Autodesk Inventor part; units mm, degrees
(part 2 of 3)
sketch "Sketch58" plane through (4600, 2900, -5000) normal (1, 0, 0) x (0, 0, -1)
  line L0 (-8412.2457, 741.5985) -> (-6687.7543, 741.5985) construction
  line L1 (-6687.7543, 741.5985) -> (-6687.7543, 358.4015) construction
  line L2 (-6687.7543, 358.4015) -> (-8412.2457, 358.4015) construction
  line L3 (-8412.2457, 358.4015) -> (-8412.2457, 741.5985) construction
  line L4 (-5750, 1200) -> (-9350, 1200) projected
  line L5 (-9350, 1200) -> (-9350, -100) projected
  line L6 (-3626.6683, 741.5985) -> (-1273.3317, 741.5985) construction
  line L7 (-1273.3317, 741.5985) -> (-1273.3317, 358.4015) construction
  line L8 (-1273.3317, 358.4015) -> (-3626.6683, 358.4015) construction
  line L9 (-3626.6683, 358.4015) -> (-3626.6683, 741.5985) construction
  line L10 (-4250, 1200) -> (-650, 1200) projected
  line L11 (-4250, -100) -> (-4250, 1200) projected
  spline S0 degree 2 poles (-8269.7933, 567.8079) (-8269.7933, 547.265) (-8286.4465, 514.2018) (-8300.4254, 504.9635) knots 0 0 0 1 2 2 2
  spline S1 degree 2 poles (-8300.4254, 504.9635) (-8311.8517, 497.7917) (-8335.312, 492.9295) (-8353.5453, 492.9295) knots 0 0 0 1 2 2 2
  line L12 (-8353.5453, 492.9295) -> (-8388.0672, 492.9295)
  line L13 (-8388.0672, 492.9295) -> (-8388.0672, 642.9295)
  line L14 (-8388.0672, 642.9295) -> (-8353.91, 642.9295)
  spline S2 degree 2 poles (-8353.91, 642.9295) (-8332.7593, 642.9295) (-8308.6912, 636.6086) (-8300.1823, 631.017) knots 0 0 0 1 2 2 2
  spline S3 degree 2 poles (-8300.1823, 631.017) (-8285.7171, 621.4141) (-8269.7933, 589.688) (-8269.7933, 567.8079) knots 0 0 0 1 2 2 2
  spline S4 degree 2 poles (-8290.5794, 568.0511) (-8290.5794, 585.312) (-8302.0056, 609.7447) (-8313.3103, 616.6734) knots 0 0 0 1 2 2 2
  spline S5 degree 2 poles (-8313.3103, 616.6734) (-8321.333, 621.4141) (-8339.4449, 625.6686) (-8352.9376, 625.6686) knots 0 0 0 1 2 2 2
  line L15 (-8352.9376, 625.6686) -> (-8368.1321, 625.6686)
  line L16 (-8368.1321, 625.6686) -> (-8368.1321, 510.1904)
  line L17 (-8368.1321, 510.1904) -> (-8352.9376, 510.1904)
  spline S6 degree 2 poles (-8352.9376, 510.1904) (-8339.688, 510.1904) (-8319.6312, 514.4449) (-8311.487, 520.158) knots 0 0 0 1 2 2 2
  spline S7 degree 2 poles (-8311.487, 520.158) (-8301.0332, 527.2083) (-8290.5794, 550.547) (-8290.5794, 568.0511) knots 0 0 0 1 2 2 2
  spline S8 degree 2 poles (-8186.8922, 504.842) (-8189.2018, 503.1402) (-8196.9813, 497.0624) (-8200.628, 495.2391) knots 0 0 0 1 2 2 2
  spline S9 degree 2 poles (-8200.628, 495.2391) (-8205.6118, 492.5648) (-8214.9716, 489.769) (-8223.4805, 489.769) knots 0 0 0 1 2 2 2
  spline S10 degree 2 poles (-8223.4805, 489.769) (-8230.4092, 489.769) (-8242.9295, 494.9959) (-8247.6701, 499.7366) knots 0 0 0 1 2 2 2
  spline S11 degree 2 poles (-8247.6701, 499.7366) (-8252.1677, 504.3558) (-8257.6377, 517.97) (-8257.6377, 525.5065) knots 0 0 0 1 2 2 2
  spline S12 degree 2 poles (-8257.6377, 525.5065) (-8257.6377, 537.1759) (-8247.7917, 553.7075) (-8237.0948, 558.4481) knots 0 0 0 1 2 2 2
  spline S13 degree 2 poles (-8237.0948, 558.4481) (-8227.6134, 562.8242) (-8201.8436, 566.1062) (-8186.8922, 566.9571) knots 0 0 0 1 2 2 2
  line L18 (-8186.8922, 566.9571) -> (-8186.8922, 570.6037)
  spline S14 degree 2 poles (-8186.8922, 570.6037) (-8186.8922, 577.1677) (-8190.9035, 585.312) (-8194.5502, 587.6216) knots 0 0 0 1 2 2 2
  spline S15 degree 2 poles (-8194.5502, 587.6216) (-8198.1969, 589.9311) (-8208.6507, 591.3898) (-8214.2423, 591.3898) knots 0 0 0 1 2 2 2
  spline S16 degree 2 poles (-8214.2423, 591.3898) (-8220.8063, 591.3898) (-8238.5535, 587.5) (-8247.427, 583.7318) knots 0 0 0 1 2 2 2
  line L19 (-8247.427, 583.7318) -> (-8248.521, 583.7318)
  line L20 (-8248.521, 583.7318) -> (-8248.521, 603.0592)
  spline S17 degree 2 poles (-8248.521, 603.0592) (-8243.2941, 604.5178) (-8223.7236, 608.1645) (-8214.1207, 608.1645) knots 0 0 0 1 2 2 2
  spline S18 degree 2 poles (-8214.1207, 608.1645) (-8202.4513, 608.1645) (-8186.5275, 604.5178) (-8180.2066, 599.7771) knots 0 0 0 1 2 2 2
  spline S19 degree 2 poles (-8180.2066, 599.7771) (-8174.0073, 595.158) (-8167.9295, 580.4498) (-8167.9295, 569.8744) knots 0 0 0 1 2 2 2
  line L21 (-8167.9295, 569.8744) -> (-8167.9295, 492.9295)
  line L22 (-8167.9295, 492.9295) -> (-8186.8922, 492.9295)
  line L23 (-8186.8922, 492.9295) -> (-8186.8922, 504.842)
  line L24 (-8186.8922, 520.6442) -> (-8186.8922, 551.8841)
  spline S20 degree 2 poles (-8186.8922, 551.8841) (-8193.6993, 551.2763) (-8214.2423, 549.2099) (-8220.6847, 547.265) knots 0 0 0 1 2 2 2
  spline S21 degree 2 poles (-8220.6847, 547.265) (-8228.2212, 544.9554) (-8238.0672, 535.3525) (-8238.0672, 526.8436) knots 0 0 0 1 2 2 2
  spline S22 degree 2 poles (-8238.0672, 526.8436) (-8238.0672, 517.1191) (-8227.1272, 507.2731) (-8216.6734, 507.2731) knots 0 0 0 1 2 2 2
  spline S23 degree 2 poles (-8216.6734, 507.2731) (-8207.7998, 507.2731) (-8193.2131, 514.9311) (-8186.8922, 520.6442) knots 0 0 0 1 2 2 2
  line L25 (-8013.675, 492.9295) -> (-8013.675, 558.0835)
  spline S24 degree 2 poles (-8013.675, 558.0835) (-8013.675, 565.863) (-8014.8906, 579.1126) (-8016.8355, 582.7593) knots 0 0 0 1 2 2 2
  spline S25 degree 2 poles (-8016.8355, 582.7593) (-8018.7804, 586.7707) (-8026.1953, 590.6605) (-8032.6377, 590.6605) knots 0 0 0 1 2 2 2
  spline S26 degree 2 poles (-8032.6377, 590.6605) (-8038.4724, 590.6605) (-8051.8436, 583.4887) (-8058.8938, 576.6815) knots 0 0 0 1 2 2 2
  spline S27 degree 2 poles (-8058.8938, 576.6815) (-8058.7723, 574.9797) (-8058.5291, 570.2391) (-8058.5291, 567.0786) knots 0 0 0 1 2 2 2
  line L26 (-8058.5291, 567.0786) -> (-8058.5291, 492.9295)
  line L27 (-8058.5291, 492.9295) -> (-8077.4919, 492.9295)
  line L28 (-8077.4919, 492.9295) -> (-8077.4919, 558.0835)
  spline S28 degree 2 poles (-8077.4919, 558.0835) (-8077.4919, 565.863) (-8078.7074, 579.1126) (-8080.6523, 582.7593) knots 0 0 0 1 2 2 2
  spline S29 degree 2 poles (-8080.6523, 582.7593) (-8082.5972, 586.7707) (-8090.0121, 590.6605) (-8096.4546, 590.6605) knots 0 0 0 1 2 2 2
  spline S30 degree 2 poles (-8096.4546, 590.6605) (-8102.5324, 590.6605) (-8116.0251, 583.0024) (-8122.346, 577.0462) knots 0 0 0 1 2 2 2
  line L29 (-8122.346, 577.0462) -> (-8122.346, 492.9295)
  line L30 (-8122.346, 492.9295) -> (-8141.3087, 492.9295)
  line L31 (-8141.3087, 492.9295) -> (-8141.3087, 605.4903)
  line L32 (-8141.3087, 605.4903) -> (-8122.346, 605.4903)
  line L33 (-8122.346, 605.4903) -> (-8122.346, 593.0916)
  spline S31 degree 2 poles (-8122.346, 593.0916) (-8114.9311, 600.5065) (-8100.3444, 608.6507) (-8091.5924, 608.6507) knots 0 0 0 1 2 2 2
  spline S32 degree 2 poles (-8091.5924, 608.6507) (-8081.6248, 608.6507) (-8066.1872, 599.534) (-8062.1758, 589.2018) knots 0 0 0 1 2 2 2
  spline S33 degree 2 poles (-8062.1758, 589.2018) (-8053.5453, 598.8047) (-8037.2569, 608.6507) (-8027.7755, 608.6507) knots 0 0 0 1 2 2 2
  spline S34 degree 2 poles (-8027.7755, 608.6507) (-8020.4821, 608.6507) (-8008.5697, 604.1532) (-8004.1936, 599.0478) knots 0 0 0 1 2 2 2
  spline S35 degree 2 poles (-8004.1936, 599.0478) (-7999.6961, 593.9425) (-7994.7123, 578.6264) (-7994.7123, 567.0786) knots 0 0 0 1 2 2 2
  line L34 (-7994.7123, 567.0786) -> (-7994.7123, 492.9295)
  line L35 (-7994.7123, 492.9295) -> (-8013.675, 492.9295)
  spline S36 degree 2 poles (-7937.4594, 489.769) (-7937.4594, 470.5632) (-7958.124, 450.3849) (-7976.2358, 450.3849) knots 0 0 0 1 2 2 2
  spline S37 degree 2 poles (-7976.2358, 450.3849) (-7979.3962, 450.3849) (-7987.1758, 450.9927) (-7990.9441, 451.6005) knots 0 0 0 1 2 2 2
  line L36 (-7990.9441, 451.6005) -> (-7990.9441, 468.6183)
  line L37 (-7990.9441, 468.6183) -> (-7989.85, 468.6183)
  spline S38 degree 2 poles (-7989.85, 468.6183) (-7987.662, 468.1321) (-7982.3136, 467.1596) (-7979.8825, 467.1596) knots 0 0 0 1 2 2 2
  spline S39 degree 2 poles (-7979.8825, 467.1596) (-7972.346, 467.1596) (-7962.5, 470.9279) (-7960.1904, 474.9392) knots 0 0 0 1 2 2 2
  spline S40 degree 2 poles (-7960.1904, 474.9392) (-7957.8808, 478.5859) (-7956.4222, 489.6475) (-7956.4222, 497.5486) knots 0 0 0 1 2 2 2
  line L38 (-7956.4222, 497.5486) -> (-7956.4222, 589.8096)
  line L39 (-7956.4222, 589.8096) -> (-7976.722, 589.8096)
  line L40 (-7976.722, 589.8096) -> (-7976.722, 605.4903)
  line L41 (-7976.722, 605.4903) -> (-7937.4594, 605.4903)
  line L42 (-7937.4594, 605.4903) -> (-7937.4594, 489.769)
  line L43 (-7937.3379, 624.2099) -> (-7958.8533, 624.2099)
  line L44 (-7958.8533, 624.2099) -> (-7958.8533, 643.9019)
  line L45 (-7958.8533, 643.9019) -> (-7937.3379, 643.9019)
  line L46 (-7937.3379, 643.9019) -> (-7937.3379, 624.2099)
  spline S41 degree 2 poles (-7847.265, 504.842) (-7849.5745, 503.1402) (-7857.3541, 497.0624) (-7861.0008, 495.2391) knots 0 0 0 1 2 2 2
  spline S42 degree 2 poles (-7861.0008, 495.2391) (-7865.9846, 492.5648) (-7875.3444, 489.769) (-7883.8533, 489.769) knots 0 0 0 1 2 2 2
  spline S43 degree 2 poles (-7883.8533, 489.769) (-7890.782, 489.769) (-7903.3022, 494.9959) (-7908.0429, 499.7366) knots 0 0 0 1 2 2 2
  spline S44 degree 2 poles (-7908.0429, 499.7366) (-7912.5405, 504.3558) (-7918.0105, 517.97) (-7918.0105, 525.5065) knots 0 0 0 1 2 2 2
  spline S45 degree 2 poles (-7918.0105, 525.5065) (-7918.0105, 537.1759) (-7908.1645, 553.7075) (-7897.4676, 558.4481) knots 0 0 0 1 2 2 2
  spline S46 degree 2 poles (-7897.4676, 558.4481) (-7887.9862, 562.8242) (-7862.2163, 566.1062) (-7847.265, 566.9571) knots 0 0 0 1 2 2 2
  line L47 (-7847.265, 566.9571) -> (-7847.265, 570.6037)
  spline S47 degree 2 poles (-7847.265, 570.6037) (-7847.265, 577.1677) (-7851.2763, 585.312) (-7854.923, 587.6216) knots 0 0 0 1 2 2 2
  spline S48 degree 2 poles (-7854.923, 587.6216) (-7858.5697, 589.9311) (-7869.0235, 591.3898) (-7874.615, 591.3898) knots 0 0 0 1 2 2 2
  spline S49 degree 2 poles (-7874.615, 591.3898) (-7881.1791, 591.3898) (-7898.9262, 587.5) (-7907.7998, 583.7318) knots 0 0 0 1 2 2 2
  line L48 (-7907.7998, 583.7318) -> (-7908.8938, 583.7318)
  line L49 (-7908.8938, 583.7318) -> (-7908.8938, 603.0592)
  spline S50 degree 2 poles (-7908.8938, 603.0592) (-7903.6669, 604.5178) (-7884.0964, 608.1645) (-7874.4935, 608.1645) knots 0 0 0 1 2 2 2
  spline S51 degree 2 poles (-7874.4935, 608.1645) (-7862.8241, 608.1645) (-7846.9003, 604.5178) (-7840.5794, 599.7771) knots 0 0 0 1 2 2 2
  spline S52 degree 2 poles (-7840.5794, 599.7771) (-7834.38, 595.158) (-7828.3022, 580.4498) (-7828.3022, 569.8744) knots 0 0 0 1 2 2 2
  line L50 (-7828.3022, 569.8744) -> (-7828.3022, 492.9295)
  line L51 (-7828.3022, 492.9295) -> (-7847.265, 492.9295)
  line L52 (-7847.265, 492.9295) -> (-7847.265, 504.842)
  line L53 (-7847.265, 520.6442) -> (-7847.265, 551.8841)
  spline S53 degree 2 poles (-7847.265, 551.8841) (-7854.0721, 551.2763) (-7874.615, 549.2099) (-7881.0575, 547.265) knots 0 0 0 1 2 2 2
  spline S54 degree 2 poles (-7881.0575, 547.265) (-7888.594, 544.9554) (-7898.44, 535.3525) (-7898.44, 526.8436) knots 0 0 0 1 2 2 2
  spline S55 degree 2 poles (-7898.44, 526.8436) (-7898.44, 517.1191) (-7887.5, 507.2731) (-7877.0462, 507.2731) knots 0 0 0 1 2 2 2
  spline S56 degree 2 poles (-7877.0462, 507.2731) (-7868.1726, 507.2731) (-7853.5859, 514.9311) (-7847.265, 520.6442) knots 0 0 0 1 2 2 2
  line L54 (-7713.3103, 492.9295) -> (-7732.2731, 492.9295)
  line L55 (-7732.2731, 492.9295) -> (-7732.2731, 557.111)
  spline S57 degree 2 poles (-7732.2731, 557.111) (-7732.2731, 564.8906) (-7733.7317, 578.2618) (-7735.9197, 582.2731) knots 0 0 0 1 2 2 2
  spline S58 degree 2 poles (-7735.9197, 582.2731) (-7738.2293, 586.5276) (-7746.4951, 590.6605) (-7753.5453, 590.6605) knots 0 0 0 1 2 2 2
  spline S59 degree 2 poles (-7753.5453, 590.6605) (-7760.5956, 590.6605) (-7775.547, 583.124) (-7782.7188, 577.0462) knots 0 0 0 1 2 2 2
  line L56 (-7782.7188, 577.0462) -> (-7782.7188, 492.9295)
  line L57 (-7782.7188, 492.9295) -> (-7801.6815, 492.9295)
  line L58 (-7801.6815, 492.9295) -> (-7801.6815, 605.4903)
  line L59 (-7801.6815, 605.4903) -> (-7782.7188, 605.4903)
  line L60 (-7782.7188, 605.4903) -> (-7782.7188, 592.97)
  spline S60 degree 2 poles (-7782.7188, 592.97) (-7774.2099, 600.628) (-7757.7998, 608.6507) (-7748.5616, 608.6507) knots 0 0 0 1 2 2 2
  spline S61 degree 2 poles (-7748.5616, 608.6507) (-7732.03, 608.6507) (-7713.3103, 586.7707) (-7713.3103, 565.9846) knots 0 0 0 1 2 2 2
  line L61 (-7713.3103, 565.9846) -> (-7713.3103, 492.9295)
  line L62 (-7525.1418, 492.9295) -> (-7629.923, 492.9295)
  line L63 (-7629.923, 492.9295) -> (-7629.923, 511.5276)
  line L64 (-7629.923, 511.5276) -> (-7549.6961, 625.1823)
  line L65 (-7549.6961, 625.1823) -> (-7626.2763, 625.1823)
  line L66 (-7626.2763, 625.1823) -> (-7626.2763, 642.9295)
  line L67 (-7626.2763, 642.9295) -> (-7527.2082, 642.9295)
  line L68 (-7527.2082, 642.9295) -> (-7527.2082, 624.9392)
  line L69 (-7527.2082, 624.9392) -> (-7608.286, 510.6767)
  line L70 (-7608.286, 510.6767) -> (-7525.1418, 510.6767)
  line L71 (-7525.1418, 510.6767) -> (-7525.1418, 492.9295)
  spline S62 degree 2 poles (-7458.0429, 490.3768) (-7485.0283, 490.3768) (-7514.688, 520.6442) (-7514.688, 548.6021) knots 0 0 0 1 2 2 2
  spline S63 degree 2 poles (-7514.688, 548.6021) (-7514.688, 576.0737) (-7485.8792, 608.6507) (-7462.662, 608.6507) knots 0 0 0 1 2 2 2
  spline S64 degree 2 poles (-7462.662, 608.6507) (-7452.2082, 608.6507) (-7436.0413, 602.5729) (-7430.0851, 596.1305) knots 0 0 0 1 2 2 2
  spline S65 degree 2 poles (-7430.0851, 596.1305) (-7424.0073, 589.688) (-7417.5648, 571.09) (-7417.5648, 557.5972) knots 0 0 0 1 2 2 2
  line L72 (-7417.5648, 557.5972) -> (-7417.5648, 547.265)
  line L73 (-7417.5648, 547.265) -> (-7495.4821, 547.265)
  spline S66 degree 2 poles (-7495.4821, 547.265) (-7495.4821, 527.6945) (-7475.7901, 506.9084) (-7458.286, 506.9084) knots 0 0 0 1 2 2 2
  spline S67 degree 2 poles (-7458.286, 506.9084) (-7452.0867, 506.9084) (-7440.0526, 509.7042) (-7435.1904, 511.8922) knots 0 0 0 1 2 2 2
  spline S68 degree 2 poles (-7435.1904, 511.8922) (-7430.0851, 514.3233) (-7423.0348, 518.5778) (-7420.7253, 520.5227) knots 0 0 0 1 2 2 2
  line L74 (-7420.7253, 520.5227) -> (-7419.6312, 520.5227)
  line L75 (-7419.6312, 520.5227) -> (-7419.6312, 499.8582)
  spline S69 degree 2 poles (-7419.6312, 499.8582) (-7422.9133, 498.5211) (-7432.8808, 494.6313) (-7436.7706, 493.5373) knots 0 0 0 1 2 2 2
  spline S70 degree 2 poles (-7436.7706, 493.5373) (-7442.2406, 491.9571) (-7451.2358, 490.3768) (-7458.0429, 490.3768) knots 0 0 0 1 2 2 2
  spline S71 degree 2 poles (-7436.0413, 561.7301) (-7436.2844, 569.3882) (-7439.4449, 580.5713) (-7442.4838, 584.3395) knots 0 0 0 1 2 2 2
  spline S72 degree 2 poles (-7442.4838, 584.3395) (-7445.7658, 588.594) (-7456.098, 593.0916) (-7463.756, 593.0916) knots 0 0 0 1 2 2 2
  spline S73 degree 2 poles (-7463.756, 593.0916) (-7471.2925, 593.0916) (-7481.8679, 588.594) (-7486.2439, 584.218) knots 0 0 0 1 2 2 2
  spline S74 degree 2 poles (-7486.2439, 584.218) (-7490.4983, 579.7204) (-7494.8744, 568.9019) (-7495.4821, 561.7301) knots 0 0 0 1 2 2 2
  line L76 (-7495.4821, 561.7301) -> (-7436.0413, 561.7301)
  line L77 (-7379.0316, 492.9295) -> (-7397.9943, 492.9295)
  line L78 (-7397.9943, 492.9295) -> (-7397.9943, 649.6151)
  line L79 (-7397.9943, 649.6151) -> (-7379.0316, 649.6151)
  line L80 (-7379.0316, 649.6151) -> (-7379.0316, 492.9295)
  spline S75 degree 2 poles (-7302.3298, 490.3768) (-7329.3152, 490.3768) (-7358.9748, 520.6442) (-7358.9748, 548.6021) knots 0 0 0 1 2 2 2
  spline S76 degree 2 poles (-7358.9748, 548.6021) (-7358.9748, 576.0737) (-7330.1661, 608.6507) (-7306.9489, 608.6507) knots 0 0 0 1 2 2 2
  spline S77 degree 2 poles (-7306.9489, 608.6507) (-7296.4951, 608.6507) (-7280.3282, 602.5729) (-7274.3719, 596.1305) knots 0 0 0 1 2 2 2
  spline S78 degree 2 poles (-7274.3719, 596.1305) (-7268.2941, 589.688) (-7261.8517, 571.09) (-7261.8517, 557.5972) knots 0 0 0 1 2 2 2
  line L81 (-7261.8517, 557.5972) -> (-7261.8517, 547.265)
  line L82 (-7261.8517, 547.265) -> (-7339.769, 547.265)
  spline S79 degree 2 poles (-7339.769, 547.265) (-7339.769, 527.6945) (-7320.077, 506.9084) (-7302.5729, 506.9084) knots 0 0 0 1 2 2 2
  spline S80 degree 2 poles (-7302.5729, 506.9084) (-7296.3736, 506.9084) (-7284.3395, 509.7042) (-7279.4773, 511.8922) knots 0 0 0 1 2 2 2
  spline S81 degree 2 poles (-7279.4773, 511.8922) (-7274.3719, 514.3233) (-7267.3217, 518.5778) (-7265.0121, 520.5227) knots 0 0 0 1 2 2 2
  line L83 (-7265.0121, 520.5227) -> (-7263.9181, 520.5227)
  line L84 (-7263.9181, 520.5227) -> (-7263.9181, 499.8582)
  spline S82 degree 2 poles (-7263.9181, 499.8582) (-7267.2001, 498.5211) (-7277.1677, 494.6313) (-7281.0575, 493.5373) knots 0 0 0 1 2 2 2
  spline S83 degree 2 poles (-7281.0575, 493.5373) (-7286.5275, 491.9571) (-7295.5227, 490.3768) (-7302.3298, 490.3768) knots 0 0 0 1 2 2 2
  spline S84 degree 2 poles (-7280.3282, 561.7301) (-7280.5713, 569.3882) (-7283.7317, 580.5713) (-7286.7706, 584.3395) knots 0 0 0 1 2 2 2
  spline S85 degree 2 poles (-7286.7706, 584.3395) (-7290.0526, 588.594) (-7300.3849, 593.0916) (-7308.0429, 593.0916) knots 0 0 0 1 2 2 2
  spline S86 degree 2 poles (-7308.0429, 593.0916) (-7315.5794, 593.0916) (-7326.1547, 588.594) (-7330.5308, 584.218) knots 0 0 0 1 2 2 2
  spline S87 degree 2 poles (-7330.5308, 584.218) (-7334.7852, 579.7204) (-7339.1612, 568.9019) (-7339.769, 561.7301) knots 0 0 0 1 2 2 2
  line L85 (-7339.769, 561.7301) -> (-7280.3282, 561.7301)
  line L86 (-7154.2747, 492.9295) -> (-7173.2374, 492.9295)
  line L87 (-7173.2374, 492.9295) -> (-7173.2374, 557.111)
  spline S88 degree 2 poles (-7173.2374, 557.111) (-7173.2374, 564.8906) (-7174.6961, 578.2618) (-7176.8841, 582.2731) knots 0 0 0 1 2 2 2
  spline S89 degree 2 poles (-7176.8841, 582.2731) (-7179.1936, 586.5276) (-7187.4594, 590.6605) (-7194.5097, 590.6605) knots 0 0 0 1 2 2 2
  spline S90 degree 2 poles (-7194.5097, 590.6605) (-7201.5599, 590.6605) (-7216.5113, 583.124) (-7223.6831, 577.0462) knots 0 0 0 1 2 2 2
  line L88 (-7223.6831, 577.0462) -> (-7223.6831, 492.9295)
  line L89 (-7223.6831, 492.9295) -> (-7242.6458, 492.9295)
  line L90 (-7242.6458, 492.9295) -> (-7242.6458, 605.4903)
  line L91 (-7242.6458, 605.4903) -> (-7223.6831, 605.4903)
  line L92 (-7223.6831, 605.4903) -> (-7223.6831, 592.97)
  spline S91 degree 2 poles (-7223.6831, 592.97) (-7215.1742, 600.628) (-7198.7641, 608.6507) (-7189.5259, 608.6507) knots 0 0 0 1 2 2 2
  spline S92 degree 2 poles (-7189.5259, 608.6507) (-7172.9943, 608.6507) (-7154.2747, 586.7707) (-7154.2747, 565.9846) knots 0 0 0 1 2 2 2
  line L93 (-7154.2747, 565.9846) -> (-7154.2747, 492.9295)
  spline S93 degree 2 poles (-7033.3265, 551.0332) (-7033.3265, 523.44) (-7060.0689, 489.769) (-7080.2471, 489.769) knots 0 0 0 1 2 2 2
  spline S94 degree 2 poles (-7080.2471, 489.769) (-7089.3638, 489.769) (-7102.3703, 494.2666) (-7108.6912, 498.1564) knots 0 0 0 1 2 2 2
  line L94 (-7108.6912, 498.1564) -> (-7109.9068, 492.9295)
  line L95 (-7109.9068, 492.9295) -> (-7127.6539, 492.9295)
  line L96 (-7127.6539, 492.9295) -> (-7127.6539, 649.6151)
  line L97 (-7127.6539, 649.6151) -> (-7108.6912, 649.6151)
  line L98 (-7108.6912, 649.6151) -> (-7108.6912, 593.6994)
  spline S95 degree 2 poles (-7108.6912, 593.6994) (-7101.5194, 600.1418) (-7084.8663, 608.6507) (-7074.2909, 608.6507) knots 0 0 0 1 2 2 2
  spline S96 degree 2 poles (-7074.2909, 608.6507) (-7055.2066, 608.6507) (-7033.3265, 578.1402) (-7033.3265, 551.0332) knots 0 0 0 1 2 2 2
  spline S97 degree 2 poles (-7052.8971, 549.5746) (-7052.8971, 569.7528) (-7065.1742, 590.6605) (-7078.7885, 590.6605) knots 0 0 0 1 2 2 2
  spline S98 degree 2 poles (-7078.7885, 590.6605) (-7086.4465, 590.6605) (-7102.2488, 583.3671) (-7108.6912, 577.7755) knots 0 0 0 1 2 2 2
  line L99 (-7108.6912, 577.7755) -> (-7108.6912, 513.2293)
  spline S99 degree 2 poles (-7108.6912, 513.2293) (-7101.5194, 509.7042) (-7090.4578, 506.7869) (-7083.8938, 506.7869) knots 0 0 0 1 2 2 2
  spline S100 degree 2 poles (-7083.8938, 506.7869) (-7069.4287, 506.7869) (-7052.8971, 527.3298) (-7052.8971, 549.5746) knots 0 0 0 1 2 2 2
  spline S101 degree 2 poles (-6950.9116, 504.842) (-6953.2212, 503.1402) (-6961.0008, 497.0624) (-6964.6475, 495.2391) knots 0 0 0 1 2 2 2
  spline S102 degree 2 poles (-6964.6475, 495.2391) (-6969.6312, 492.5648) (-6978.9911, 489.769) (-6987.5, 489.769) knots 0 0 0 1 2 2 2
  spline S103 degree 2 poles (-6987.5, 489.769) (-6994.4287, 489.769) (-7006.9489, 494.9959) (-7011.6896, 499.7366) knots 0 0 0 1 2 2 2
  spline S104 degree 2 poles (-7011.6896, 499.7366) (-7016.1872, 504.3558) (-7021.6572, 517.97) (-7021.6572, 525.5065) knots 0 0 0 1 2 2 2
  spline S105 degree 2 poles (-7021.6572, 525.5065) (-7021.6572, 537.1759) (-7011.8112, 553.7075) (-7001.1142, 558.4481) knots 0 0 0 1 2 2 2
  spline S106 degree 2 poles (-7001.1142, 558.4481) (-6991.6329, 562.8242) (-6965.863, 566.1062) (-6950.9116, 566.9571) knots 0 0 0 1 2 2 2
  line L100 (-6950.9116, 566.9571) -> (-6950.9116, 570.6037)
  spline S107 degree 2 poles (-6950.9116, 570.6037) (-6950.9116, 577.1677) (-6954.923, 585.312) (-6958.5697, 587.6216) knots 0 0 0 1 2 2 2
  spline S108 degree 2 poles (-6958.5697, 587.6216) (-6962.2163, 589.9311) (-6972.6701, 591.3898) (-6978.2617, 591.3898) knots 0 0 0 1 2 2 2
  spline S109 degree 2 poles (-6978.2617, 591.3898) (-6984.8257, 591.3898) (-7002.5729, 587.5) (-7011.4465, 583.7318) knots 0 0 0 1 2 2 2
  line L101 (-7011.4465, 583.7318) -> (-7012.5405, 583.7318)
  line L102 (-7012.5405, 583.7318) -> (-7012.5405, 603.0592)
  spline S110 degree 2 poles (-7012.5405, 603.0592) (-7007.3136, 604.5178) (-6987.7431, 608.1645) (-6978.1402, 608.1645) knots 0 0 0 1 2 2 2
  spline S111 degree 2 poles (-6978.1402, 608.1645) (-6966.4708, 608.1645) (-6950.547, 604.5178) (-6944.2261, 599.7771) knots 0 0 0 1 2 2 2
  spline S112 degree 2 poles (-6944.2261, 599.7771) (-6938.0267, 595.158) (-6931.9489, 580.4498) (-6931.9489, 569.8744) knots 0 0 0 1 2 2 2
  line L103 (-6931.9489, 569.8744) -> (-6931.9489, 492.9295)
  line L104 (-6931.9489, 492.9295) -> (-6950.9116, 492.9295)
  line L105 (-6950.9116, 492.9295) -> (-6950.9116, 504.842)
  line L106 (-6950.9116, 520.6442) -> (-6950.9116, 551.8841)
  spline S113 degree 2 poles (-6950.9116, 551.8841) (-6957.7188, 551.2763) (-6978.2617, 549.2099) (-6984.7042, 547.265) knots 0 0 0 1 2 2 2
  spline S114 degree 2 poles (-6984.7042, 547.265) (-6992.2406, 544.9554) (-7002.0867, 535.3525) (-7002.0867, 526.8436) knots 0 0 0 1 2 2 2
  spline S115 degree 2 poles (-7002.0867, 526.8436) (-7002.0867, 517.1191) (-6991.1466, 507.2731) (-6980.6928, 507.2731) knots 0 0 0 1 2 2 2
  spline S116 degree 2 poles (-6980.6928, 507.2731) (-6971.8193, 507.2731) (-6957.2325, 514.9311) (-6950.9116, 520.6442) knots 0 0 0 1 2 2 2
  spline S117 degree 2 poles (-6811.0008, 551.0332) (-6811.0008, 523.44) (-6837.7431, 489.769) (-6857.9214, 489.769) knots 0 0 0 1 2 2 2
  spline S118 degree 2 poles (-6857.9214, 489.769) (-6867.0381, 489.769) (-6880.0445, 494.2666) (-6886.3654, 498.1564) knots 0 0 0 1 2 2 2
  line L107 (-6886.3654, 498.1564) -> (-6887.581, 492.9295)
  line L108 (-6887.581, 492.9295) -> (-6905.3282, 492.9295)
  line L109 (-6905.3282, 492.9295) -> (-6905.3282, 649.6151)
  line L110 (-6905.3282, 649.6151) -> (-6886.3654, 649.6151)
  line L111 (-6886.3654, 649.6151) -> (-6886.3654, 593.6994)
  spline S119 degree 2 poles (-6886.3654, 593.6994) (-6879.1936, 600.1418) (-6862.5405, 608.6507) (-6851.9651, 608.6507) knots 0 0 0 1 2 2 2
  spline S120 degree 2 poles (-6851.9651, 608.6507) (-6832.8808, 608.6507) (-6811.0008, 578.1402) (-6811.0008, 551.0332) knots 0 0 0 1 2 2 2
  spline S121 degree 2 poles (-6830.5713, 549.5746) (-6830.5713, 569.7528) (-6842.8484, 590.6605) (-6856.4627, 590.6605) knots 0 0 0 1 2 2 2
  spline S122 degree 2 poles (-6856.4627, 590.6605) (-6864.1207, 590.6605) (-6879.923, 583.3671) (-6886.3654, 577.7755) knots 0 0 0 1 2 2 2
  line L112 (-6886.3654, 577.7755) -> (-6886.3654, 513.2293)
  spline S123 degree 2 poles (-6886.3654, 513.2293) (-6879.1936, 509.7042) (-6868.1321, 506.7869) (-6861.568, 506.7869) knots 0 0 0 1 2 2 2
  spline S124 degree 2 poles (-6861.568, 506.7869) (-6847.1029, 506.7869) (-6830.5713, 527.3298) (-6830.5713, 549.5746) knots 0 0 0 1 2 2 2
  spline S125 degree 2 poles (-6728.5859, 504.842) (-6730.8954, 503.1402) (-6738.675, 497.0624) (-6742.3217, 495.2391) knots 0 0 0 1 2 2 2
  spline S126 degree 2 poles (-6742.3217, 495.2391) (-6747.3055, 492.5648) (-6756.6653, 489.769) (-6765.1742, 489.769) knots 0 0 0 1 2 2 2
  spline S127 degree 2 poles (-6765.1742, 489.769) (-6772.1029, 489.769) (-6784.6231, 494.9959) (-6789.3638, 499.7366) knots 0 0 0 1 2 2 2
  spline S128 degree 2 poles (-6789.3638, 499.7366) (-6793.8614, 504.3558) (-6799.3314, 517.97) (-6799.3314, 525.5065) knots 0 0 0 1 2 2 2
  spline S129 degree 2 poles (-6799.3314, 525.5065) (-6799.3314, 537.1759) (-6789.4854, 553.7075) (-6778.7885, 558.4481) knots 0 0 0 1 2 2 2
  spline S130 degree 2 poles (-6778.7885, 558.4481) (-6769.3071, 562.8242) (-6743.5372, 566.1062) (-6728.5859, 566.9571) knots 0 0 0 1 2 2 2
  line L113 (-6728.5859, 566.9571) -> (-6728.5859, 570.6037)
  spline S131 degree 2 poles (-6728.5859, 570.6037) (-6728.5859, 577.1677) (-6732.5972, 585.312) (-6736.2439, 587.6216) knots 0 0 0 1 2 2 2
  spline S132 degree 2 poles (-6736.2439, 587.6216) (-6739.8906, 589.9311) (-6750.3444, 591.3898) (-6755.9359, 591.3898) knots 0 0 0 1 2 2 2
  spline S133 degree 2 poles (-6755.9359, 591.3898) (-6762.5, 591.3898) (-6780.2471, 587.5) (-6789.1207, 583.7318) knots 0 0 0 1 2 2 2
  line L114 (-6789.1207, 583.7318) -> (-6790.2147, 583.7318)
  line L115 (-6790.2147, 583.7318) -> (-6790.2147, 603.0592)
  spline S134 degree 2 poles (-6790.2147, 603.0592) (-6784.9878, 604.5178) (-6765.4173, 608.1645) (-6755.8144, 608.1645) knots 0 0 0 1 2 2 2
  spline S135 degree 2 poles (-6755.8144, 608.1645) (-6744.145, 608.1645) (-6728.2212, 604.5178) (-6721.9003, 599.7771) knots 0 0 0 1 2 2 2
  spline S136 degree 2 poles (-6721.9003, 599.7771) (-6715.7009, 595.158) (-6709.6231, 580.4498) (-6709.6231, 569.8744) knots 0 0 0 1 2 2 2
  line L116 (-6709.6231, 569.8744) -> (-6709.6231, 492.9295)
  line L117 (-6709.6231, 492.9295) -> (-6728.5859, 492.9295)
  line L118 (-6728.5859, 492.9295) -> (-6728.5859, 504.842)
  line L119 (-6728.5859, 520.6442) -> (-6728.5859, 551.8841)
  spline S137 degree 2 poles (-6728.5859, 551.8841) (-6735.393, 551.2763) (-6755.9359, 549.2099) (-6762.3784, 547.265) knots 0 0 0 1 2 2 2
  spline S138 degree 2 poles (-6762.3784, 547.265) (-6769.9149, 544.9554) (-6779.7609, 535.3525) (-6779.7609, 526.8436) knots 0 0 0 1 2 2 2
  spline S139 degree 2 poles (-6779.7609, 526.8436) (-6779.7609, 517.1191) (-6768.8209, 507.2731) (-6758.3671, 507.2731) knots 0 0 0 1 2 2 2
  spline S140 degree 2 poles (-6758.3671, 507.2731) (-6749.4935, 507.2731) (-6734.9068, 514.9311) (-6728.5859, 520.6442) knots 0 0 0 1 2 2 2
  spline S141 degree 2 poles (-3169.7933, 567.8079) (-3169.7933, 547.265) (-3186.4465, 514.2018) (-3200.4254, 504.9635) knots 0 0 0 1 2 2 2
  spline S142 degree 2 poles (-3200.4254, 504.9635) (-3211.8517, 497.7917) (-3235.312, 492.9295) (-3253.5453, 492.9295) knots 0 0 0 1 2 2 2
  line L120 (-3253.5453, 492.9295) -> (-3288.0672, 492.9295)
  line L121 (-3288.0672, 492.9295) -> (-3288.0672, 642.9295)
  line L122 (-3288.0672, 642.9295) -> (-3253.91, 642.9295)
  spline S143 degree 2 poles (-3253.91, 642.9295) (-3232.7593, 642.9295) (-3208.6912, 636.6086) (-3200.1823, 631.017) knots 0 0 0 1 2 2 2
  spline S144 degree 2 poles (-3200.1823, 631.017) (-3185.7171, 621.4141) (-3169.7933, 589.688) (-3169.7933, 567.8079) knots 0 0 0 1 2 2 2
  spline S145 degree 2 poles (-3190.5794, 568.0511) (-3190.5794, 585.312) (-3202.0056, 609.7447) (-3213.3103, 616.6734) knots 0 0 0 1 2 2 2
  spline S146 degree 2 poles (-3213.3103, 616.6734) (-3221.333, 621.4141) (-3239.4449, 625.6686) (-3252.9376, 625.6686) knots 0 0 0 1 2 2 2
  line L123 (-3252.9376, 625.6686) -> (-3268.1321, 625.6686)
  line L124 (-3268.1321, 625.6686) -> (-3268.1321, 510.1904)
  line L125 (-3268.1321, 510.1904) -> (-3252.9376, 510.1904)
  spline S147 degree 2 poles (-3252.9376, 510.1904) (-3239.688, 510.1904) (-3219.6312, 514.4449) (-3211.487, 520.158) knots 0 0 0 1 2 2 2
  spline S148 degree 2 poles (-3211.487, 520.158) (-3201.0332, 527.2083) (-3190.5794, 550.547) (-3190.5794, 568.0511) knots 0 0 0 1 2 2 2
  spline S149 degree 2 poles (-3086.8922, 504.842) (-3089.2018, 503.1402) (-3096.9813, 497.0624) (-3100.628, 495.2391) knots 0 0 0 1 2 2 2
  spline S150 degree 2 poles (-3100.628, 495.2391) (-3105.6118, 492.5648) (-3114.9716, 489.769) (-3123.4805, 489.769) knots 0 0 0 1 2 2 2
  spline S151 degree 2 poles (-3123.4805, 489.769) (-3130.4092, 489.769) (-3142.9295, 494.9959) (-3147.6701, 499.7366) knots 0 0 0 1 2 2 2
  spline S152 degree 2 poles (-3147.6701, 499.7366) (-3152.1677, 504.3558) (-3157.6377, 517.97) (-3157.6377, 525.5065) knots 0 0 0 1 2 2 2
  spline S153 degree 2 poles (-3157.6377, 525.5065) (-3157.6377, 537.1759) (-3147.7917, 553.7075) (-3137.0948, 558.4481) knots 0 0 0 1 2 2 2
  spline S154 degree 2 poles (-3137.0948, 558.4481) (-3127.6134, 562.8242) (-3101.8436, 566.1062) (-3086.8922, 566.9571) knots 0 0 0 1 2 2 2
  line L126 (-3086.8922, 566.9571) -> (-3086.8922, 570.6037)
  spline S155 degree 2 poles (-3086.8922, 570.6037) (-3086.8922, 577.1677) (-3090.9035, 585.312) (-3094.5502, 587.6216) knots 0 0 0 1 2 2 2
  spline S156 degree 2 poles (-3094.5502, 587.6216) (-3098.1969, 589.9311) (-3108.6507, 591.3898) (-3114.2423, 591.3898) knots 0 0 0 1 2 2 2
  spline S157 degree 2 poles (-3114.2423, 591.3898) (-3120.8063, 591.3898) (-3138.5535, 587.5) (-3147.427, 583.7318) knots 0 0 0 1 2 2 2
  line L127 (-3147.427, 583.7318) -> (-3148.521, 583.7318)
  line L128 (-3148.521, 583.7318) -> (-3148.521, 603.0592)
  spline S158 degree 2 poles (-3148.521, 603.0592) (-3143.2941, 604.5178) (-3123.7236, 608.1645) (-3114.1207, 608.1645) knots 0 0 0 1 2 2 2
  spline S159 degree 2 poles (-3114.1207, 608.1645) (-3102.4513, 608.1645) (-3086.5275, 604.5178) (-3080.2066, 599.7771) knots 0 0 0 1 2 2 2
  spline S160 degree 2 poles (-3080.2066, 599.7771) (-3074.0073, 595.158) (-3067.9295, 580.4498) (-3067.9295, 569.8744) knots 0 0 0 1 2 2 2
  line L129 (-3067.9295, 569.8744) -> (-3067.9295, 492.9295)
  line L130 (-3067.9295, 492.9295) -> (-3086.8922, 492.9295)
  line L131 (-3086.8922, 492.9295) -> (-3086.8922, 504.842)
  line L132 (-3086.8922, 520.6442) -> (-3086.8922, 551.8841)
  spline S161 degree 2 poles (-3086.8922, 551.8841) (-3093.6993, 551.2763) (-3114.2423, 549.2099) (-3120.6847, 547.265) knots 0 0 0 1 2 2 2
  spline S162 degree 2 poles (-3120.6847, 547.265) (-3128.2212, 544.9554) (-3138.0672, 535.3525) (-3138.0672, 526.8436) knots 0 0 0 1 2 2 2
  spline S163 degree 2 poles (-3138.0672, 526.8436) (-3138.0672, 517.1191) (-3127.1272, 507.2731) (-3116.6734, 507.2731) knots 0 0 0 1 2 2 2
  spline S164 degree 2 poles (-3116.6734, 507.2731) (-3107.7998, 507.2731) (-3093.2131, 514.9311) (-3086.8922, 520.6442) knots 0 0 0 1 2 2 2
  line L133 (-2913.675, 492.9295) -> (-2913.675, 558.0835)
  spline S165 degree 2 poles (-2913.675, 558.0835) (-2913.675, 565.863) (-2914.8906, 579.1126) (-2916.8355, 582.7593) knots 0 0 0 1 2 2 2
  spline S166 degree 2 poles (-2916.8355, 582.7593) (-2918.7804, 586.7707) (-2926.1953, 590.6605) (-2932.6377, 590.6605) knots 0 0 0 1 2 2 2
  spline S167 degree 2 poles (-2932.6377, 590.6605) (-2938.4724, 590.6605) (-2951.8436, 583.4887) (-2958.8938, 576.6815) knots 0 0 0 1 2 2 2
  spline S168 degree 2 poles (-2958.8938, 576.6815) (-2958.7723, 574.9797) (-2958.5291, 570.2391) (-2958.5291, 567.0786) knots 0 0 0 1 2 2 2
  line L134 (-2958.5291, 567.0786) -> (-2958.5291, 492.9295)
  line L135 (-2958.5291, 492.9295) -> (-2977.4919, 492.9295)
  line L136 (-2977.4919, 492.9295) -> (-2977.4919, 558.0835)
  spline S169 degree 2 poles (-2977.4919, 558.0835) (-2977.4919, 565.863) (-2978.7074, 579.1126) (-2980.6523, 582.7593) knots 0 0 0 1 2 2 2
  spline S170 degree 2 poles (-2980.6523, 582.7593) (-2982.5972, 586.7707) (-2990.0121, 590.6605) (-2996.4546, 590.6605) knots 0 0 0 1 2 2 2
  spline S171 degree 2 poles (-2996.4546, 590.6605) (-3002.5324, 590.6605) (-3016.0251, 583.0024) (-3022.346, 577.0462) knots 0 0 0 1 2 2 2
  line L137 (-3022.346, 577.0462) -> (-3022.346, 492.9295)
  line L138 (-3022.346, 492.9295) -> (-3041.3087, 492.9295)
  line L139 (-3041.3087, 492.9295) -> (-3041.3087, 605.4903)
  line L140 (-3041.3087, 605.4903) -> (-3022.346, 605.4903)
  line L141 (-3022.346, 605.4903) -> (-3022.346, 593.0916)
  spline S172 degree 2 poles (-3022.346, 593.0916) (-3014.9311, 600.5065) (-3000.3444, 608.6507) (-2991.5924, 608.6507) knots 0 0 0 1 2 2 2
  spline S173 degree 2 poles (-2991.5924, 608.6507) (-2981.6248, 608.6507) (-2966.1872, 599.534) (-2962.1758, 589.2018) knots 0 0 0 1 2 2 2
  spline S174 degree 2 poles (-2962.1758, 589.2018) (-2953.5453, 598.8047) (-2937.2569, 608.6507) (-2927.7755, 608.6507) knots 0 0 0 1 2 2 2
  spline S175 degree 2 poles (-2927.7755, 608.6507) (-2920.4821, 608.6507) (-2908.5697, 604.1532) (-2904.1936, 599.0478) knots 0 0 0 1 2 2 2
  spline S176 degree 2 poles (-2904.1936, 599.0478) (-2899.6961, 593.9425) (-2894.7123, 578.6264) (-2894.7123, 567.0786) knots 0 0 0 1 2 2 2
  line L142 (-2894.7123, 567.0786) -> (-2894.7123, 492.9295)
  line L143 (-2894.7123, 492.9295) -> (-2913.675, 492.9295)
  spline S177 degree 2 poles (-2837.4594, 489.769) (-2837.4594, 470.5632) (-2858.124, 450.3849) (-2876.2358, 450.3849) knots 0 0 0 1 2 2 2
  spline S178 degree 2 poles (-2876.2358, 450.3849) (-2879.3962, 450.3849) (-2887.1758, 450.9927) (-2890.9441, 451.6005) knots 0 0 0 1 2 2 2
  line L144 (-2890.9441, 451.6005) -> (-2890.9441, 468.6183)
  line L145 (-2890.9441, 468.6183) -> (-2889.85, 468.6183)
  spline S179 degree 2 poles (-2889.85, 468.6183) (-2887.662, 468.1321) (-2882.3136, 467.1596) (-2879.8825, 467.1596) knots 0 0 0 1 2 2 2
  spline S180 degree 2 poles (-2879.8825, 467.1596) (-2872.346, 467.1596) (-2862.5, 470.9279) (-2860.1904, 474.9392) knots 0 0 0 1 2 2 2
  spline S181 degree 2 poles (-2860.1904, 474.9392) (-2857.8808, 478.5859) (-2856.4222, 489.6475) (-2856.4222, 497.5486) knots 0 0 0 1 2 2 2
  line L146 (-2856.4222, 497.5486) -> (-2856.4222, 589.8096)
  line L147 (-2856.4222, 589.8096) -> (-2876.722, 589.8096)
  line L148 (-2876.722, 589.8096) -> (-2876.722, 605.4903)
  line L149 (-2876.722, 605.4903) -> (-2837.4594, 605.4903)
  line L150 (-2837.4594, 605.4903) -> (-2837.4594, 489.769)
  line L151 (-2837.3379, 624.2099) -> (-2858.8533, 624.2099)
  line L152 (-2858.8533, 624.2099) -> (-2858.8533, 643.9019)
  line L153 (-2858.8533, 643.9019) -> (-2837.3379, 643.9019)
  line L154 (-2837.3379, 643.9019) -> (-2837.3379, 624.2099)
  spline S182 degree 2 poles (-2747.265, 504.842) (-2749.5745, 503.1402) (-2757.3541, 497.0624) (-2761.0008, 495.2391) knots 0 0 0 1 2 2 2
  spline S183 degree 2 poles (-2761.0008, 495.2391) (-2765.9846, 492.5648) (-2775.3444, 489.769) (-2783.8533, 489.769) knots 0 0 0 1 2 2 2
  spline S184 degree 2 poles (-2783.8533, 489.769) (-2790.782, 489.769) (-2803.3022, 494.9959) (-2808.0429, 499.7366) knots 0 0 0 1 2 2 2
  spline S185 degree 2 poles (-2808.0429, 499.7366) (-2812.5405, 504.3558) (-2818.0105, 517.97) (-2818.0105, 525.5065) knots 0 0 0 1 2 2 2
  spline S186 degree 2 poles (-2818.0105, 525.5065) (-2818.0105, 537.1759) (-2808.1645, 553.7075) (-2797.4676, 558.4481) knots 0 0 0 1 2 2 2
  spline S187 degree 2 poles (-2797.4676, 558.4481) (-2787.9862, 562.8242) (-2762.2163, 566.1062) (-2747.265, 566.9571) knots 0 0 0 1 2 2 2
  line L155 (-2747.265, 566.9571) -> (-2747.265, 570.6037)
  spline S188 degree 2 poles (-2747.265, 570.6037) (-2747.265, 577.1677) (-2751.2763, 585.312) (-2754.923, 587.6216) knots 0 0 0 1 2 2 2
  spline S189 degree 2 poles (-2754.923, 587.6216) (-2758.5697, 589.9311) (-2769.0235, 591.3898) (-2774.615, 591.3898) knots 0 0 0 1 2 2 2
  spline S190 degree 2 poles (-2774.615, 591.3898) (-2781.1791, 591.3898) (-2798.9262, 587.5) (-2807.7998, 583.7318) knots 0 0 0 1 2 2 2
  line L156 (-2807.7998, 583.7318) -> (-2808.8938, 583.7318)
  line L157 (-2808.8938, 583.7318) -> (-2808.8938, 603.0592)
  spline S191 degree 2 poles (-2808.8938, 603.0592) (-2803.6669, 604.5178) (-2784.0964, 608.1645) (-2774.4935, 608.1645) knots 0 0 0 1 2 2 2
  spline S192 degree 2 poles (-2774.4935, 608.1645) (-2762.8241, 608.1645) (-2746.9003, 604.5178) (-2740.5794, 599.7771) knots 0 0 0 1 2 2 2
  spline S193 degree 2 poles (-2740.5794, 599.7771) (-2734.38, 595.158) (-2728.3022, 580.4498) (-2728.3022, 569.8744) knots 0 0 0 1 2 2 2
  line L158 (-2728.3022, 569.8744) -> (-2728.3022, 492.9295)
  line L159 (-2728.3022, 492.9295) -> (-2747.265, 492.9295)
  line L160 (-2747.265, 492.9295) -> (-2747.265, 504.842)
  line L161 (-2747.265, 520.6442) -> (-2747.265, 551.8841)
  spline S194 degree 2 poles (-2747.265, 551.8841) (-2754.0721, 551.2763) (-2774.615, 549.2099) (-2781.0575, 547.265) knots 0 0 0 1 2 2 2
  spline S195 degree 2 poles (-2781.0575, 547.265) (-2788.594, 544.9554) (-2798.44, 535.3525) (-2798.44, 526.8436) knots 0 0 0 1 2 2 2
  spline S196 degree 2 poles (-2798.44, 526.8436) (-2798.44, 517.1191) (-2787.5, 507.2731) (-2777.0462, 507.2731) knots 0 0 0 1 2 2 2
  spline S197 degree 2 poles (-2777.0462, 507.2731) (-2768.1726, 507.2731) (-2753.5859, 514.9311) (-2747.265, 520.6442) knots 0 0 0 1 2 2 2
  line L162 (-2613.3103, 492.9295) -> (-2632.2731, 492.9295)
  line L163 (-2632.2731, 492.9295) -> (-2632.2731, 557.111)
  spline S198 degree 2 poles (-2632.2731, 557.111) (-2632.2731, 564.8906) (-2633.7317, 578.2618) (-2635.9197, 582.2731) knots 0 0 0 1 2 2 2
  spline S199 degree 2 poles (-2635.9197, 582.2731) (-2638.2293, 586.5276) (-2646.4951, 590.6605) (-2653.5453, 590.6605) knots 0 0 0 1 2 2 2
  spline S200 degree 2 poles (-2653.5453, 590.6605) (-2660.5956, 590.6605) (-2675.547, 583.124) (-2682.7188, 577.0462) knots 0 0 0 1 2 2 2
  line L164 (-2682.7188, 577.0462) -> (-2682.7188, 492.9295)
  line L165 (-2682.7188, 492.9295) -> (-2701.6815, 492.9295)
  line L166 (-2701.6815, 492.9295) -> (-2701.6815, 605.4903)
  line L167 (-2701.6815, 605.4903) -> (-2682.7188, 605.4903)
  line L168 (-2682.7188, 605.4903) -> (-2682.7188, 592.97)
  spline S201 degree 2 poles (-2682.7188, 592.97) (-2674.2099, 600.628) (-2657.7998, 608.6507) (-2648.5616, 608.6507) knots 0 0 0 1 2 2 2
  spline S202 degree 2 poles (-2648.5616, 608.6507) (-2632.03, 608.6507) (-2613.3103, 586.7707) (-2613.3103, 565.9846) knots 0 0 0 1 2 2 2
  line L169 (-2613.3103, 565.9846) -> (-2613.3103, 492.9295)
  line L170 (-2425.1418, 492.9295) -> (-2529.923, 492.9295)
  line L171 (-2529.923, 492.9295) -> (-2529.923, 511.5276)
  line L172 (-2529.923, 511.5276) -> (-2449.6961, 625.1823)
  line L173 (-2449.6961, 625.1823) -> (-2526.2763, 625.1823)
  line L174 (-2526.2763, 625.1823) -> (-2526.2763, 642.9295)
  line L175 (-2526.2763, 642.9295) -> (-2427.2082, 642.9295)
  line L176 (-2427.2082, 642.9295) -> (-2427.2082, 624.9392)
  line L177 (-2427.2082, 624.9392) -> (-2508.286, 510.6767)
  line L178 (-2508.286, 510.6767) -> (-2425.1418, 510.6767)
  line L179 (-2425.1418, 510.6767) -> (-2425.1418, 492.9295)
  spline S203 degree 2 poles (-2358.0429, 490.3768) (-2385.0283, 490.3768) (-2414.688, 520.6442) (-2414.688, 548.6021) knots 0 0 0 1 2 2 2
  spline S204 degree 2 poles (-2414.688, 548.6021) (-2414.688, 576.0737) (-2385.8792, 608.6507) (-2362.662, 608.6507) knots 0 0 0 1 2 2 2
  spline S205 degree 2 poles (-2362.662, 608.6507) (-2352.2082, 608.6507) (-2336.0413, 602.5729) (-2330.0851, 596.1305) knots 0 0 0 1 2 2 2
  spline S206 degree 2 poles (-2330.0851, 596.1305) (-2324.0073, 589.688) (-2317.5648, 571.09) (-2317.5648, 557.5972) knots 0 0 0 1 2 2 2
  line L180 (-2317.5648, 557.5972) -> (-2317.5648, 547.265)
  line L181 (-2317.5648, 547.265) -> (-2395.4821, 547.265)
  spline S207 degree 2 poles (-2395.4821, 547.265) (-2395.4821, 527.6945) (-2375.7901, 506.9084) (-2358.286, 506.9084) knots 0 0 0 1 2 2 2
  spline S208 degree 2 poles (-2358.286, 506.9084) (-2352.0867, 506.9084) (-2340.0526, 509.7042) (-2335.1904, 511.8922) knots 0 0 0 1 2 2 2
  spline S209 degree 2 poles (-2335.1904, 511.8922) (-2330.0851, 514.3233) (-2323.0348, 518.5778) (-2320.7253, 520.5227) knots 0 0 0 1 2 2 2
  line L182 (-2320.7253, 520.5227) -> (-2319.6312, 520.5227)
  line L183 (-2319.6312, 520.5227) -> (-2319.6312, 499.8582)
  spline S210 degree 2 poles (-2319.6312, 499.8582) (-2322.9133, 498.5211) (-2332.8808, 494.6313) (-2336.7706, 493.5373) knots 0 0 0 1 2 2 2
  spline S211 degree 2 poles (-2336.7706, 493.5373) (-2342.2406, 491.9571) (-2351.2358, 490.3768) (-2358.0429, 490.3768) knots 0 0 0 1 2 2 2
  spline S212 degree 2 poles (-2336.0413, 561.7301) (-2336.2844, 569.3882) (-2339.4449, 580.5713) (-2342.4838, 584.3395) knots 0 0 0 1 2 2 2
  spline S213 degree 2 poles (-2342.4838, 584.3395) (-2345.7658, 588.594) (-2356.098, 593.0916) (-2363.756, 593.0916) knots 0 0 0 1 2 2 2
  spline S214 degree 2 poles (-2363.756, 593.0916) (-2371.2925, 593.0916) (-2381.8679, 588.594) (-2386.2439, 584.218) knots 0 0 0 1 2 2 2
  spline S215 degree 2 poles (-2386.2439, 584.218) (-2390.4983, 579.7204) (-2394.8744, 568.9019) (-2395.4821, 561.7301) knots 0 0 0 1 2 2 2
  line L184 (-2395.4821, 561.7301) -> (-2336.0413, 561.7301)
  line L185 (-2279.0316, 492.9295) -> (-2297.9943, 492.9295)
  line L186 (-2297.9943, 492.9295) -> (-2297.9943, 649.6151)
  line L187 (-2297.9943, 649.6151) -> (-2279.0316, 649.6151)
  line L188 (-2279.0316, 649.6151) -> (-2279.0316, 492.9295)
  spline S216 degree 2 poles (-2202.3298, 490.3768) (-2229.3152, 490.3768) (-2258.9748, 520.6442) (-2258.9748, 548.6021) knots 0 0 0 1 2 2 2
  spline S217 degree 2 poles (-2258.9748, 548.6021) (-2258.9748, 576.0737) (-2230.1661, 608.6507) (-2206.9489, 608.6507) knots 0 0 0 1 2 2 2
  spline S218 degree 2 poles (-2206.9489, 608.6507) (-2196.4951, 608.6507) (-2180.3282, 602.5729) (-2174.3719, 596.1305) knots 0 0 0 1 2 2 2
  spline S219 degree 2 poles (-2174.3719, 596.1305) (-2168.2941, 589.688) (-2161.8517, 571.09) (-2161.8517, 557.5972) knots 0 0 0 1 2 2 2
  line L189 (-2161.8517, 557.5972) -> (-2161.8517, 547.265)
  line L190 (-2161.8517, 547.265) -> (-2239.769, 547.265)
  spline S220 degree 2 poles (-2239.769, 547.265) (-2239.769, 527.6945) (-2220.077, 506.9084) (-2202.5729, 506.9084) knots 0 0 0 1 2 2 2
  spline S221 degree 2 poles (-2202.5729, 506.9084) (-2196.3736, 506.9084) (-2184.3395, 509.7042) (-2179.4773, 511.8922) knots 0 0 0 1 2 2 2
  spline S222 degree 2 poles (-2179.4773, 511.8922) (-2174.3719, 514.3233) (-2167.3217, 518.5778) (-2165.0121, 520.5227) knots 0 0 0 1 2 2 2
  line L191 (-2165.0121, 520.5227) -> (-2163.9181, 520.5227)
  line L192 (-2163.9181, 520.5227) -> (-2163.9181, 499.8582)
  spline S223 degree 2 poles (-2163.9181, 499.8582) (-2167.2001, 498.5211) (-2177.1677, 494.6313) (-2181.0575, 493.5373) knots 0 0 0 1 2 2 2
  spline S224 degree 2 poles (-2181.0575, 493.5373) (-2186.5275, 491.9571) (-2195.5227, 490.3768) (-2202.3298, 490.3768) knots 0 0 0 1 2 2 2
  spline S225 degree 2 poles (-2180.3282, 561.7301) (-2180.5713, 569.3882) (-2183.7317, 580.5713) (-2186.7706, 584.3395) knots 0 0 0 1 2 2 2
  spline S226 degree 2 poles (-2186.7706, 584.3395) (-2190.0526, 588.594) (-2200.3849, 593.0916) (-2208.0429, 593.0916) knots 0 0 0 1 2 2 2
  spline S227 degree 2 poles (-2208.0429, 593.0916) (-2215.5794, 593.0916) (-2226.1547, 588.594) (-2230.5308, 584.218) knots 0 0 0 1 2 2 2
  spline S228 degree 2 poles (-2230.5308, 584.218) (-2234.7852, 579.7204) (-2239.1612, 568.9019) (-2239.769, 561.7301) knots 0 0 0 1 2 2 2
  line L193 (-2239.769, 561.7301) -> (-2180.3282, 561.7301)
  line L194 (-2054.2747, 492.9295) -> (-2073.2374, 492.9295)
  line L195 (-2073.2374, 492.9295) -> (-2073.2374, 557.111)
  spline S229 degree 2 poles (-2073.2374, 557.111) (-2073.2374, 564.8906) (-2074.6961, 578.2618) (-2076.8841, 582.2731) knots 0 0 0 1 2 2 2
  spline S230 degree 2 poles (-2076.8841, 582.2731) (-2079.1936, 586.5276) (-2087.4594, 590.6605) (-2094.5097, 590.6605) knots 0 0 0 1 2 2 2
  spline S231 degree 2 poles (-2094.5097, 590.6605) (-2101.5599, 590.6605) (-2116.5113, 583.124) (-2123.6831, 577.0462) knots 0 0 0 1 2 2 2
  line L196 (-2123.6831, 577.0462) -> (-2123.6831, 492.9295)
  line L197 (-2123.6831, 492.9295) -> (-2142.6458, 492.9295)
  line L198 (-2142.6458, 492.9295) -> (-2142.6458, 605.4903)
  line L199 (-2142.6458, 605.4903) -> (-2123.6831, 605.4903)
  line L200 (-2123.6831, 605.4903) -> (-2123.6831, 592.97)
  spline S232 degree 2 poles (-2123.6831, 592.97) (-2115.1742, 600.628) (-2098.7641, 608.6507) (-2089.5259, 608.6507) knots 0 0 0 1 2 2 2
  spline S233 degree 2 poles (-2089.5259, 608.6507) (-2072.9943, 608.6507) (-2054.2747, 586.7707) (-2054.2747, 565.9846) knots 0 0 0 1 2 2 2
  line L201 (-2054.2747, 565.9846) -> (-2054.2747, 492.9295)
  spline S234 degree 2 poles (-1933.3265, 551.0332) (-1933.3265, 523.44) (-1960.0689, 489.769) (-1980.2471, 489.769) knots 0 0 0 1 2 2 2
  spline S235 degree 2 poles (-1980.2471, 489.769) (-1989.3638, 489.769) (-2002.3703, 494.2666) (-2008.6912, 498.1564) knots 0 0 0 1 2 2 2
  line L202 (-2008.6912, 498.1564) -> (-2009.9068, 492.9295)
  line L203 (-2009.9068, 492.9295) -> (-2027.6539, 492.9295)
  line L204 (-2027.6539, 492.9295) -> (-2027.6539, 649.6151)
  line L205 (-2027.6539, 649.6151) -> (-2008.6912, 649.6151)
  line L206 (-2008.6912, 649.6151) -> (-2008.6912, 593.6994)
  spline S236 degree 2 poles (-2008.6912, 593.6994) (-2001.5194, 600.1418) (-1984.8663, 608.6507) (-1974.2909, 608.6507) knots 0 0 0 1 2 2 2
  spline S237 degree 2 poles (-1974.2909, 608.6507) (-1955.2066, 608.6507) (-1933.3265, 578.1402) (-1933.3265, 551.0332) knots 0 0 0 1 2 2 2
  spline S238 degree 2 poles (-1952.8971, 549.5746) (-1952.8971, 569.7528) (-1965.1742, 590.6605) (-1978.7885, 590.6605) knots 0 0 0 1 2 2 2
  spline S239 degree 2 poles (-1978.7885, 590.6605) (-1986.4465, 590.6605) (-2002.2488, 583.3671) (-2008.6912, 577.7755) knots 0 0 0 1 2 2 2
  line L207 (-2008.6912, 577.7755) -> (-2008.6912, 513.2293)
  spline S240 degree 2 poles (-2008.6912, 513.2293) (-2001.5194, 509.7042) (-1990.4578, 506.7869) (-1983.8938, 506.7869) knots 0 0 0 1 2 2 2
  spline S241 degree 2 poles (-1983.8938, 506.7869) (-1969.4287, 506.7869) (-1952.8971, 527.3298) (-1952.8971, 549.5746) knots 0 0 0 1 2 2 2
  spline S242 degree 2 poles (-1850.9116, 504.842) (-1853.2212, 503.1402) (-1861.0008, 497.0624) (-1864.6475, 495.2391) knots 0 0 0 1 2 2 2
  spline S243 degree 2 poles (-1864.6475, 495.2391) (-1869.6312, 492.5648) (-1878.9911, 489.769) (-1887.5, 489.769) knots 0 0 0 1 2 2 2
  spline S244 degree 2 poles (-1887.5, 489.769) (-1894.4287, 489.769) (-1906.9489, 494.9959) (-1911.6896, 499.7366) knots 0 0 0 1 2 2 2
  spline S245 degree 2 poles (-1911.6896, 499.7366) (-1916.1872, 504.3558) (-1921.6572, 517.97) (-1921.6572, 525.5065) knots 0 0 0 1 2 2 2
  spline S246 degree 2 poles (-1921.6572, 525.5065) (-1921.6572, 537.1759) (-1911.8112, 553.7075) (-1901.1142, 558.4481) knots 0 0 0 1 2 2 2
  spline S247 degree 2 poles (-1901.1142, 558.4481) (-1891.6329, 562.8242) (-1865.863, 566.1062) (-1850.9116, 566.9571) knots 0 0 0 1 2 2 2
  line L208 (-1850.9116, 566.9571) -> (-1850.9116, 570.6037)
  spline S248 degree 2 poles (-1850.9116, 570.6037) (-1850.9116, 577.1677) (-1854.923, 585.312) (-1858.5697, 587.6216) knots 0 0 0 1 2 2 2
  spline S249 degree 2 poles (-1858.5697, 587.6216) (-1862.2163, 589.9311) (-1872.6701, 591.3898) (-1878.2617, 591.3898) knots 0 0 0 1 2 2 2
  spline S250 degree 2 poles (-1878.2617, 591.3898) (-1884.8257, 591.3898) (-1902.5729, 587.5) (-1911.4465, 583.7318) knots 0 0 0 1 2 2 2
  line L209 (-1911.4465, 583.7318) -> (-1912.5405, 583.7318)
  line L210 (-1912.5405, 583.7318) -> (-1912.5405, 603.0592)
  spline S251 degree 2 poles (-1912.5405, 603.0592) (-1907.3136, 604.5178) (-1887.7431, 608.1645) (-1878.1402, 608.1645) knots 0 0 0 1 2 2 2
  spline S252 degree 2 poles (-1878.1402, 608.1645) (-1866.4708, 608.1645) (-1850.547, 604.5178) (-1844.2261, 599.7771) knots 0 0 0 1 2 2 2
  spline S253 degree 2 poles (-1844.2261, 599.7771) (-1838.0267, 595.158) (-1831.9489, 580.4498) (-1831.9489, 569.8744) knots 0 0 0 1 2 2 2
  line L211 (-1831.9489, 569.8744) -> (-1831.9489, 492.9295)
  line L212 (-1831.9489, 492.9295) -> (-1850.9116, 492.9295)
  line L213 (-1850.9116, 492.9295) -> (-1850.9116, 504.842)
  line L214 (-1850.9116, 520.6442) -> (-1850.9116, 551.8841)
  spline S254 degree 2 poles (-1850.9116, 551.8841) (-1857.7188, 551.2763) (-1878.2617, 549.2099) (-1884.7042, 547.265) knots 0 0 0 1 2 2 2
  spline S255 degree 2 poles (-1884.7042, 547.265) (-1892.2406, 544.9554) (-1902.0867, 535.3525) (-1902.0867, 526.8436) knots 0 0 0 1 2 2 2
  spline S256 degree 2 poles (-1902.0867, 526.8436) (-1902.0867, 517.1191) (-1891.1466, 507.2731) (-1880.6928, 507.2731) knots 0 0 0 1 2 2 2
  spline S257 degree 2 poles (-1880.6928, 507.2731) (-1871.8193, 507.2731) (-1857.2325, 514.9311) (-1850.9116, 520.6442) knots 0 0 0 1 2 2 2
  spline S258 degree 2 poles (-1711.0008, 551.0332) (-1711.0008, 523.44) (-1737.7431, 489.769) (-1757.9214, 489.769) knots 0 0 0 1 2 2 2
  spline S259 degree 2 poles (-1757.9214, 489.769) (-1767.0381, 489.769) (-1780.0445, 494.2666) (-1786.3654, 498.1564) knots 0 0 0 1 2 2 2
  line L215 (-1786.3654, 498.1564) -> (-1787.581, 492.9295)
  line L216 (-1787.581, 492.9295) -> (-1805.3282, 492.9295)
  line L217 (-1805.3282, 492.9295) -> (-1805.3282, 649.6151)
  line L218 (-1805.3282, 649.6151) -> (-1786.3654, 649.6151)
  line L219 (-1786.3654, 649.6151) -> (-1786.3654, 593.6994)
  spline S260 degree 2 poles (-1786.3654, 593.6994) (-1779.1936, 600.1418) (-1762.5405, 608.6507) (-1751.9651, 608.6507) knots 0 0 0 1 2 2 2
  spline S261 degree 2 poles (-1751.9651, 608.6507) (-1732.8808, 608.6507) (-1711.0008, 578.1402) (-1711.0008, 551.0332) knots 0 0 0 1 2 2 2